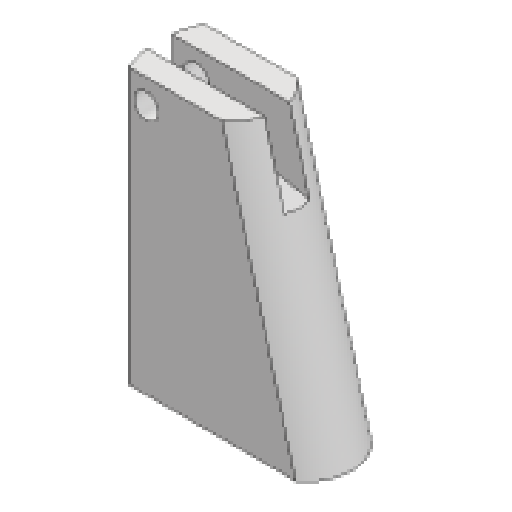
# Autodesk Inventor part: wedge
Saved by Autodesk Inventor 2023 (Build 270158000, 158)
## iProperties
Created: 2022-10-23
Part Number: wedge
Material: Generic
Document SubType Name: Modeling
Designer: deli
Density: 1 g/cm^3
Appearance: Default
Author: deli
Autodesk Inventor part; units mm, degrees
ref_plane "YZ Plane" through (0, 0, 0) normal (1, 0, 0) x (0, 1, 0)
ref_plane "XZ Plane" through (0, 0, 0) normal (0, 1, 0) x (-1, 0, 0)
ref_plane "XY Plane" through (0, 0, 0) normal (0, 0, 1) x (1, 0, 0)
sketch "Sketch1" plane through (0, 0, 0) normal (0, 0, 1) x (1, 0, 0)
  line L0 (-11.177, 13.2143) -> (-11.177, -30.7857)
  line L1 (-11.177, -30.7857) -> (19.823, -30.7857)
  line L2 (19.823, -30.7857) -> (8.0332, 13.2143)
  line L3 (8.0332, 13.2143) -> (-11.177, 13.2143)
  circle A0 centre (-7.177, 9.2143) radius 2
  line L4 (-11.177, -30.7857) -> (-11.177, 9.2143) construction
  line L5 (-11.177, -34.7857) -> (-3.177, -34.7857) construction
  line L6 (-3.177, -34.7857) -> (-3.177, 9.2143) construction
  arc A1 (-3.177, 9.2143) -> (-11.177, 9.2143) centre (-7.177, 9.2143) ccw construction
  line L7 (-12.3103, -7.3446) -> (19.4397, -7.3446) construction
  line L8 (3.5647, -7.3446) -> (3.5647, -29.2883) construction
  line L9 (19.4397, -7.3446) -> (19.8228, -29.2883) construction
  line L10 (-17.3867, 7.2951) -> (25.318, -1.7821) construction
  circle A2 centre (24.2015, -7.2615) radius 4.7625 construction
  circle A3 centre (21.3465, -29.2617) radius 1.524 construction
  line L11 (-12.6933, -29.2883) -> (19.8228, -29.2883) construction
  circle A4 centre (-14.2171, -29.2617) radius 1.524 construction
  line L12 (-12.3103, -7.3446) -> (-12.6933, -29.2883) construction
  line L13 (-11.177, -30.7857) -> (-15.177, -30.7857) construction
  line L14 (-15.177, -30.7857) -> (-11.177, -34.7857) construction
  circle A5 centre (-14.2171, -29.2617) radius 40.1639 construction
  point P0 (0, 0)
  dimension "d52" = 9.525
  dimension "d53" = 3.048
  dimension "d0" = 31
  dimension "d1" = 4
  dimension "d4" = 4
  dimension "d5" = 4
  dimension "d7" = 8
  dimension "d8" = 40
  dimension "d9" = 44
  dimension "d11" = 31.75
  dimension "d13" = 21.9437
  dimension "d54" = 32.5161
  dimension "d56" = 4
  dimension "d58" = 4
  dimension "d60" = 35.5636
  dimension "d61" = 3.0401
  dimension "d63" = 75
  dimension "d64" = 0
  dimension "d66" = 78
  constraints: 30 end point, 4 perpendicular, 3 tangent, 2 centre point, 2 horizontal, 2 midpoint, 2 parallel, 2 point on circle, 2 vertical, 1 coincident, 1 concentric, 1 point on line, 15 other
  measures "d0" distance of L0.end L1.end
  measures "d1" diameter of A0
  measures "d4" distance from line of L0 A0.centre
  measures "d5" distance from line of L3 A0.centre
  measures "d7" distance between parallel lines of L6 L4
  measures "d8" distance from line of L1 A0.centre
  measures "d9" distance of L5.end L6.end
  measures "d11" distance of L7.end L7.start
  measures "d13" distance of L8.end L8.start
  measures "d54" distance of L9.end L11.start
  measures "d56" distance of L4.start L13.end
  measures "d58" distance between parallel lines of L5 L13
  measures "d60" distance of point (21.347, -29.262) point (-14.217, -29.262)
  measures "d61" horizontal distance of L0.end point (-14.217, -29.262)
  measures "d63" angle of L2 L1
  measures "d64" distance from line of L0 L4.start
  measures "d66" angle of L6 L10
extrude "Extrusion1" add sketch "Sketch1" along normal blind 4
sketch "Sketch2" plane through (0, 0, 4) normal (0, 0, 1) x (1, 0, 0)
  line L0 (8.0332, 13.2143) -> (-11.177, 13.2143) projected
  line L1 (-4.0448, 13.2143) -> (7.257, -32.5429)
  line L2 (19.823, -30.7857) -> (8.0332, 13.2143) projected
  circle A0 centre (-7.177, 9.2143) radius 2 projected
  line L3 (-9.7939, 3.1281) -> (-1.4688, -30.5779) construction
  line L4 (-1.4688, -30.5779) -> (-11.177, -32.9758) construction
  line L5 (-11.177, -32.9758) -> (-10.2178, -36.8591) construction
  line L6 (-10.2178, -36.8591) -> (7.257, -32.5429) construction
  line L7 (-11.177, 13.2143) -> (-11.177, -30.7857) construction
  line L8 (-11.177, -30.7857) -> (19.823, -30.7857) projected
  line L9 (-11.177, 5.0813) -> (10.0266, 5.7751)
  line L10 (-11.177, 8.0198) -> (10.6693, 3.3762)
  line L11 (-9.9165, 15.9306) -> (8.3455, 12.0489)
  line L12 (-10.5708, 11.1043) -> (8.432, 11.7261)
  point P0 (0, 0)
  point P1 (6.823, -30.7857)
  point P2 (-3.5801, 11.333)
  point P3 (-2.2955, 6.132)
  dimension "d22" = 4
  dimension "d23" = 8
  dimension "d24" = 4
  dimension "d25" = 10
  dimension "d26" = 40
  dimension "d31" = 4
  dimension "d32" = 78
  dimension "d33" = 2
  dimension "d34" = 78
  dimension "d35" = 2
  dimension "d36" = 6
  constraints: 18 end point, 8 point on line, 5 parallel, 1 perpendicular
  measures "d22" distance from line of L1 A0.centre
  measures "d23" distance between parallel lines of L1 L3
  measures "d24" distance between parallel lines of L6 L4
  measures "d25" distance of L3.end L4.end
  measures "d26" distance from line of L4 A0.centre
  measures "d31" distance from line of A0.centre L9
  measures "d32" angle of L9 L1
  measures "d33" distance from line of A0.centre L10
  measures "d34" angle of L7 L10
  measures "d35" distance from line of L12 A0.centre
  measures "d36" distance from line of A0.centre L11
extrude "Extrusion2" add sketch "Sketch2" along normal blind 4 contours L10 L9 L1 | L2 L8 L1 L9 L10
sketch "Sketch3" plane through (0, 0, 8) normal (0, 0, 1) x (1, 0, 0)
  line L0 (-11.177, -30.7857) -> (19.823, -30.7857) projected
  line L1 (-11.177, 13.2143) -> (-11.177, -30.7857) projected
  line L2 (8.0332, 13.2143) -> (-11.177, 13.2143) projected
  line L3 (19.823, -30.7857) -> (8.0332, 13.2143) projected
  circle A0 centre (-7.177, 9.2143) radius 2 projected
  point P0 (0, 0)
extrude "Extrusion3" add sketch "Sketch3" along normal blind 4
sketch "Sketch5" plane through (19.823, -30.7857, 12) normal (0.9659258, 0.258819, 0) x (0, 0, -1)
  line L0 (12, 0) -> (0, 0) projected
  line L1 (12, 0) -> (12, 45.5522) projected
  line L2 (0, 0) -> (12, 0)
  line L3 (12, 0) -> (12, 4.3237)
  line L4 (12, 4.3237) -> (0, 4.3237)
  line L5 (0, 4.3237) -> (0, 0)
  point P0 (12, 34.8673)
  constraints: 8 end point, 2 parallel, 1 horizontal, 1 perpendicular, 1 point on line
extrude "Extrusion5" add sketch "Sketch5" along normal blind 4
sketch "Sketch6" plane through (19.823, -30.7857, 0) normal (0.258819, -0.9659258, 0) x (0.9659258, 0.258819, 0)
  circle A0 centre (-7.5, 6) radius 7.5
  line L0 (0, 0) -> (0, 12) projected
  line L1 (-3, 12) -> (-3, 0)
  line L2 (-29.9437, 12) -> (0, 12) projected
  line L3 (-29.9437, 0) -> (0, 0) projected
  line L4 (-15.4151, 7.5875) -> (4.9413, 7.5875) projected
  line L5 (0, 0) -> (0, 12) projected
  line L6 (0, 0) -> (4, 0) projected
  line L7 (4, 12) -> (4, 0) projected
  line L8 (0, 12) -> (4, 12) projected
  point P0 (-11.1796, 0)
  point P1 (0, 6)
  point P2 (0, 0)
  point P3 (0, 12)
  dimension "d43" = 6
  dimension "d44" = 12
  dimension "d45" = 3
  constraints: 2 end point, 2 point on circle, 1 centre point, 1 tangent, 1 vertical
  measures "d43" vertical distance of L0.start A0.centre
  measures "d44" distance of L1.start L1.end
  measures "d45" distance between parallel lines of L0 L1
extrude "Extrusion6" cut sketch "Sketch6" against normal blind 50 contours A0 L0 L3 | L0 L4 L7 L6 | A0 L4 L0 | A0 L2 L0 L4 | L0 L8 L7 L4
sketch "Sketch7" plane through (-11.177, -30.7857, 0) normal (0, -1, 0) x (1, 0, 0)
  circle A0 centre (15.5, 6) radius 15.5
  line L0 (0, 12) -> (27.8942, 12) projected
  ellipse E0 centre (23.2354, 6) end of major axis (15.4709, 6) minor radius 7.5 (27.8942, 0) -> (27.8942, 12) ccw projected
  circle A1 centre (15.5, 6) radius 19.8481
  point P0 (11.177, 0)
  dimension "d48" = 31
  dimension "d49" = 6
  constraints: 2 centre point, 1 coincident, 2 other
  measures "d48" diameter of A0
  measures "d49" distance from line of A0.centre L0
extrude "Extrusion7" cut sketch "Sketch7" against normal blind 50
body "Solid1"
